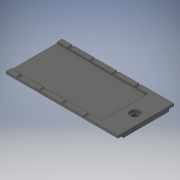
# Autodesk Inventor part: TNS_Greiferbacke_MA_Jun_T2
Saved by Autodesk Inventor 2017 (Build 210142000, 142)
## iProperties
Created: 2018-03-14
Part Number: TNS_Greiferbacke_MA_Jun_T2
Material: Generic
Document SubType Name: Modeling
Designer: uoehq
Density: 1 g/cm^3
Appearance: Gray
Author: uoehq
Autodesk Inventor part; units mm, degrees
ref_plane "YZ Plane" through (0, 0, 0) normal (1, 0, 0) x (0, 1, 0)
ref_plane "XZ Plane" through (0, 0, 0) normal (0, 1, 0) x (-1, 0, 0)
ref_plane "XY Plane" through (0, 0, 0) normal (0, 0, 1) x (1, 0, 0)
sketch "Sketch1" plane through (0, 0, 0) normal (0, 0, 1) x (1, 0, 0)
  line L0 (0, 0) -> (100, 0)
  line L1 (100, 0) -> (100, -50)
  line L2 (100, -50) -> (0, -50)
  line L3 (0, -50) -> (0, 0)
  dimension "d2" = 100
  dimension "d3" = 50
  constraints: 8 end point, 2 parallel, 1 horizontal, 1 perpendicular
  measures "d2" distance of L0.start L0.end
  measures "d3" distance of L2.end L0.start
extrude "Extrusion1" add sketch "Sketch1" along normal blind 4
sketch "Sketch2" plane through (0, 0, 0) normal (0, 0, -1) x (-1, 0, 0)
  line L0 (0, 0) -> (0, -50) projected
  line L1 (0, -50) -> (-100, -50)
  line L2 (-100, -50) -> (-100, -45.5)
  line L3 (-100, -45.5) -> (0, -45.5)
  line L4 (0, -45.5) -> (0, -50)
  line L5 (0, 0) -> (-100, 0)
  line L6 (-100, 0) -> (-100, -4.5)
  line L7 (-100, -4.5) -> (0, -4.5)
  line L8 (0, -4.5) -> (0, 0)
  line L9 (-100, -50) -> (-100, 0) projected
  dimension "d6" = 4.5
  dimension "d7" = 4.5
  dimension "d16" = 0
  dimension "d17" = 0
  constraints: 16 end point, 4 parallel, 2 horizontal, 2 perpendicular
  measures "d6" distance between parallel lines of L1 L3
  measures "d7" distance between parallel lines of L5 L7
  measures "d16" distance between parallel lines of L9 L6
  measures "d17" distance between parallel lines of L9 L2
extrude "Extrusion2" cut sketch "Sketch2" against normal blind 2 contours L0 L7 L6 L5 | L0 L1 L2 L3
fillet "Fillet1" radius 0.5 2 edges at (50, -45.5, 0) (50, -4.5, 0)
sketch "Sketch3" plane through (0, 0, 4) normal (0, 0, 1) x (1, 0, 0)
  line L0 (0, -45) -> (0, -5) projected
  line L1 (0, -4.5) -> (81, -4.5)
  line L2 (81, -4.5) -> (81, -45.5)
  line L3 (81, -45.5) -> (0, -45.5)
  line L4 (0, -45.5) -> (0, -4.5)
  line L5 (100, 0) -> (0, 0) projected
  dimension "d11" = 81
  dimension "d12" = 41
  dimension "d13" = 4.5
  constraints: 8 end point, 2 parallel, 1 horizontal, 1 perpendicular, 1 point on line
  measures "d11" distance of L1.start L1.end
  measures "d12" distance of L1.end L2.end
  measures "d13" distance between parallel lines of L5 L1
extrude "Extrusion3" cut sketch "Sketch3" against normal blind 1
sketch "Sketch5" plane through (0, 0, 4) normal (0, 0, 1) x (1, 0, 0)
  line L0 (100, 0) -> (0, 0) projected
  line L1 (100, -50) -> (100, 0) projected
  point P0 (90, -25)
  dimension "d37" = 25
  dimension "d38" = 10
  measures "d37" distance from line of L0 point (90, -25)
  measures "d38" distance from line of L1 point (90, -25)
hole "Hole1" at (90, -25, 4) direction (0, 0, -1) diameter 4.5 end through all counterbore diameter 8 counterbore depth 2
hole "Hole2" at (10, -50, 4) direction (0, 1, 0) diameter 2 end through all
pattern_linear "Rectangular Pattern1" count 4 spacing 20 along (1, 0, 0) of "Hole2"
body "Solid1"
